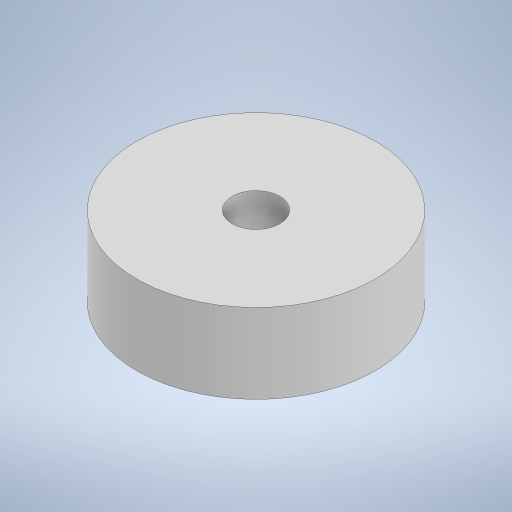
# Autodesk Inventor part: 1. ring
Saved by Autodesk Inventor 2024 (Build 280153000, 153)
## iProperties
Created: 2024-02-22
Part Number: 1. ring
Material: Generic
Document SubType Name: Modeling
Designer: evmgm
Density: 1 g/cm^3
Appearance: Default
Author: evmgm
Autodesk Inventor part; units mm, degrees
ref_plane "YZ Plane" through (0, 0, 0) normal (1, 0, 0) x (0, 1, 0)
ref_plane "XZ Plane" through (0, 0, 0) normal (0, 1, 0) x (-1, 0, 0)
ref_plane "XY Plane" through (0, 0, 0) normal (0, 0, 1) x (1, 0, 0)
sketch "Sketch1" plane through (0, 0, 0) normal (0, 1, 0) x (-1, 0, 0)
  circle A0 centre (0, 0) radius 6
  circle A1 centre (0, 0) radius 30
  dimension "d0" = 12
  dimension "d1" = 60
  constraints: 2 centre point, 2 coincident
  measures "d0" diameter of A0
  measures "d1" diameter of A1
extrude "Extrusion1" add sketch "Sketch1" along normal blind 20 contours A0 | A1
hole "Hole1" at (0, 0, 0) direction (0, 1, 0) diameter 12 end through all countersink diameter 25 countersink angle 61.2
body "Solid1"
